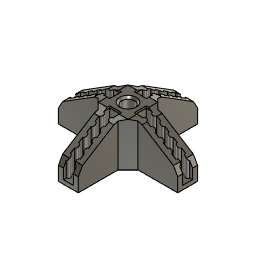
QuadAdapters4 (Autodesk Fusion 360 design; units mm, degrees)
Autodesk Fusion 360 part; units mm, degrees
sketch "Sketch1" plane through (0, 0, 0) normal (0, 0, 1) x (1, 0, 0)
  line L0 (0, 0) -> (0, 50)
  line L1 (0, 50) -> (10, 50)
  line L2 (10, 50) -> (10, 0)
  line L3 (10, 0) -> (60, 0)
  line L4 (60, 0) -> (60, -10)
  line L5 (60, -10) -> (10, -10)
  line L6 (10, -10) -> (10, -60)
  line L7 (10, -60) -> (0, -60)
  line L8 (0, -60) -> (0, -10)
  line L9 (0, -10) -> (-50, -10)
  line L10 (-50, -10) -> (-50, 0)
  line L11 (-50, 0) -> (0, 0)
  line L12 (-5, 5) -> (-5, 55)
  line L13 (-5, 55) -> (15, 55)
  line L14 (15, 55) -> (15, 5)
  line L15 (15, 5) -> (65, 5)
  line L16 (65, 5) -> (65, -15)
  line L17 (65, -15) -> (15, -15)
  line L18 (15, -15) -> (15, -65)
  line L19 (15, -65) -> (-5, -65)
  line L20 (-5, -65) -> (-5, -15)
  line L21 (-5, -15) -> (-55, -15)
  line L22 (-55, -15) -> (-55, 5)
  line L23 (-55, 5) -> (-5, 5)
  line L24 (0, 55) -> (0, -65)
  line L25 (10, -65) -> (10, 55)
  line L26 (-55, 0) -> (65, 0)
  line L27 (65, -10) -> (-55, -10)
  circle A0 centre (0, 50) radius 2.1
  circle A1 centre (10, 50) radius 2.1
  circle A2 centre (0, 41.6667) radius 2.1
  circle A3 centre (10, 41.6667) radius 2.1
  circle A4 centre (0, 33.3333) radius 2.1
  circle A5 centre (10, 33.3333) radius 2.1
  circle A6 centre (0, 25) radius 2.1
  circle A7 centre (10, 25) radius 2.1
  circle A8 centre (0, 16.6667) radius 2.1
  circle A9 centre (10, 16.6667) radius 2.1
  circle A10 centre (0, 8.3333) radius 2.1
  circle A11 centre (10, 8.3333) radius 2.1
  circle A12 centre (0, 0) radius 2.1
  circle A13 centre (10, 0) radius 2.1
  line L28 (-68.0742, -5) -> (73.3109, -5)
  line L29 (5, 62.6678) -> (5, -70)
  circle A14 centre (0, -18.3333) radius 2.1
  circle A15 centre (10, -43.3333) radius 2.1
  line L30 (0, -60) -> (10, -60)
  circle A16 centre (0, -43.3333) radius 2.1
  circle A17 centre (0, -26.6667) radius 2.1
  line L31 (10, -60) -> (10, -10)
  circle A18 centre (0, -10) radius 2.1
  circle A19 centre (10, -35) radius 2.1
  circle A20 centre (0, -35) radius 2.1
  circle A21 centre (10, -51.6667) radius 2.1
  line L32 (0, -10) -> (0, -60)
  circle A22 centre (0, -51.6667) radius 2.1
  circle A23 centre (10, -26.6667) radius 2.1
  line L33 (-5, -15) -> (-5, -65)
  circle A24 centre (10, -10) radius 2.1
  circle A25 centre (0, -60) radius 2.1
  circle A26 centre (10, -18.3333) radius 2.1
  circle A27 centre (10, -60) radius 2.1
  circle A28 centre (-41.6667, -10) radius 2.1
  circle A29 centre (0, 0) radius 2.1
  circle A30 centre (-8.3333, -10) radius 2.1
  line L34 (-50, 0) -> (0, 0)
  circle A31 centre (-25, 0) radius 2.1
  circle A32 centre (-50, -10) radius 2.1
  circle A33 centre (-16.6667, -10) radius 2.1
  line L35 (-50, -10) -> (-50, 0)
  circle A34 centre (0, -10) radius 2.1
  circle A35 centre (-25, -10) radius 2.1
  circle A36 centre (-8.3333, 0) radius 2.1
  circle A37 centre (-33.3333, -10) radius 2.1
  circle A38 centre (-16.6667, 0) radius 2.1
  line L36 (0, -10) -> (-50, -10)
  circle A39 centre (-50, 0) radius 2.1
  circle A40 centre (-33.3333, 0) radius 2.1
  circle A41 centre (-41.6667, 0) radius 2.1
  line L37 (-55, -15) -> (-55, 5)
  circle A42 centre (10, -51.6667) radius 2.1
  circle A43 centre (0, -10) radius 2.1
  circle A44 centre (10, -18.3333) radius 2.1
  line L38 (0, -60) -> (0, -10)
  circle A45 centre (0, -35) radius 2.1
  circle A46 centre (10, -60) radius 2.1
  circle A47 centre (10, -26.6667) radius 2.1
  line L39 (10, -60) -> (0, -60)
  circle A48 centre (10, -10) radius 2.1
  circle A49 centre (10, -35) radius 2.1
  circle A50 centre (0, -18.3333) radius 2.1
  circle A51 centre (10, -43.3333) radius 2.1
  circle A52 centre (0, -26.6667) radius 2.1
  line L40 (10, -10) -> (10, -60)
  circle A53 centre (0, -60) radius 2.1
  circle A54 centre (0, -43.3333) radius 2.1
  circle A55 centre (0, -51.6667) radius 2.1
  line L41 (15, -65) -> (-5, -65)
  circle A56 centre (51.6667, 0) radius 2.1
  circle A57 centre (10, -10) radius 2.1
  circle A58 centre (18.3333, 0) radius 2.1
  line L42 (60, -10) -> (10, -10)
  circle A59 centre (35, -10) radius 2.1
  circle A60 centre (60, 0) radius 2.1
  circle A61 centre (26.6667, 0) radius 2.1
  line L43 (60, 0) -> (60, -10)
  circle A62 centre (10, 0) radius 2.1
  circle A63 centre (35, 0) radius 2.1
  circle A64 centre (18.3333, -10) radius 2.1
  circle A65 centre (43.3333, 0) radius 2.1
  circle A66 centre (26.6667, -10) radius 2.1
  line L44 (10, 0) -> (60, 0)
  circle A67 centre (60, -10) radius 2.1
  circle A68 centre (43.3333, -10) radius 2.1
  circle A69 centre (51.6667, -10) radius 2.1
  line L45 (65, 5) -> (65, -15)
  line L46 (0, 0) -> (-8.3333, 0)
  line L47 (-8.3333, 0) -> (-8.3333, -10)
  line L48 (-8.3333, -10) -> (0, -10)
  line L49 (0, -10) -> (0, 0)
  line L50 (18.3333, 0) -> (10, 0)
  line L51 (10, 0) -> (10, -10)
  line L52 (10, -10) -> (18.3333, -10)
  line L53 (18.3333, -10) -> (18.3333, 0)
  line L54 (0, 8.3333) -> (10, 8.3333)
  line L55 (10, 8.3333) -> (10, 0)
  line L56 (10, 0) -> (0, 0)
  line L57 (0, 0) -> (0, 8.3333)
  line L58 (0, -10) -> (10, -10)
  line L59 (10, -10) -> (10, -18.3333)
  line L60 (10, -18.3333) -> (0, -18.3333)
  line L61 (0, -18.3333) -> (0, -10)
  point P0 (0, -65)
  point P1 (10, -65)
  point P2 (0, -10)
  point P3 (0, -10)
  point P4 (5, -5)
  point P5 (0, -10)
  point P6 (-55, -10)
  point P7 (-5, 5)
  point P8 (-55, 0)
  point P9 (5, -5)
  point P10 (0, -10)
  point P11 (-5, -15)
  point P12 (10, -10)
  point P13 (10, -65)
  point P14 (-5, -15)
  point P15 (0, -65)
  point P16 (5, -5)
  point P17 (10, -10)
  point P18 (15, -15)
  point P19 (10, 0)
  point P20 (65, 0)
  point P21 (15, -15)
  point P22 (65, -10)
  point P23 (5, -5)
  point P24 (10, 0)
  point P25 (15, 5)
  dimension "d1" = 10
  dimension "d2" = 50
  dimension "d3" = 10
  dimension "d4" = 50
  dimension "d5" = 50
  dimension "d6" = -5
  dimension "d7" = 4.2
  dimension "d8" = 4.2
  dimension "d11" = 0
  dimension "d12" = -50
  dimension "d14" = 360
  constraint coincident L0.start L11.end
  constraint vertical L0
  constraint perpendicular L0 L1
  constraint perpendicular L1 L2
  constraint perpendicular L0 L3
  constraint perpendicular L3 L4
  constraint perpendicular L4 L5
  constraint perpendicular L5 L6
  constraint perpendicular L6 L7
  constraint perpendicular L7 L8
  constraint perpendicular L8 L9
  constraint perpendicular L7 L10
  constraint perpendicular L0 L11
  constraint coincident L13 L24.start
  constraint coincident L19 P15
  constraint perpendicular L19 L24
  constraint coincident L19 P13
  constraint coincident L13 L25.end
  constraint perpendicular L13 L25
  constraint coincident L22 P8
  constraint coincident L16 P20
  constraint perpendicular L16 L26
  constraint coincident L16 P22
  constraint coincident L22 P6
  constraint perpendicular L22 L27
  constraint coincident L0.end L1.start
  constraint coincident L1.end L2.start
  constraint perpendicular L22 L28
  constraint perpendicular L26 L29
  constraint symmetric L0.start L28 P10
  constraint symmetric L0.end L28 L7.end
  constraint symmetric L1.end L28 L6.end
  constraint symmetric P24 L28 P17
  constraint symmetric P7 L28 P11
  constraint symmetric L12.end L28 L19.end
  constraint symmetric L24.start L28 P15
  constraint symmetric L25.end L28 P13
  constraint symmetric A0 L28 A25
  constraint symmetric A1 L28 A27
  constraint symmetric A2 L28 A22
  constraint symmetric A3 L28 A21
  constraint symmetric A4 L28 A16
  constraint symmetric A5 L28 A15
  constraint symmetric A6 L28 A20
  constraint symmetric A7 L28 A19
  constraint symmetric A8 L28 A17
  constraint symmetric A9 L28 A23
  constraint symmetric A10 L28 A14
  constraint symmetric A11 L28 A26
  constraint symmetric A12 L28 A18
  constraint symmetric A13 L28 A24
  constraint coincident L28 P23
  constraint coincident L29 P23
  constraint horizontal L46
  constraint vertical L47
  constraint horizontal L48
  constraint vertical L49
  constraint coincident A30.centre L47.end
  constraint horizontal L50
  constraint vertical L51
  constraint horizontal L52
  constraint vertical L53
  constraint coincident P17 P12
  constraint coincident A58.centre L50.start
  constraint horizontal L54
  constraint vertical L55
  constraint horizontal L56
  constraint vertical L57
  constraint coincident P24 P19
  constraint coincident A10.centre L54.start
  constraint horizontal L58
  constraint vertical L59
  constraint horizontal L60
  constraint vertical L61
  constraint coincident A26.centre A44.centre
  measures "d1" distance of L0.end L1.end
  measures "d2" distance of P24 L3.end
  measures "d3" distance of L3.end L4.end
  measures "d4" distance of P17 L6.end
  measures "d5" distance of P5 L9.end
  measures "d7" diameter of A0
  measures "d8" diameter of A1
extrude "Extrude1" add sketch "Sketch1" along normal blind 45 contours L0 L11 L24 L26 A12 A29 L34 L46 L57 | L11 L24 L26 A12 A29 L34 L46 L49 | L24 L26 A12 A29 L49 L56 | L0 L24 L26 A12 A29 L56 L57 | L0 L11 L12 L13 L22 L23 L24 L26 A0 A2 A4 A6 A8 A10 A12 A29 L34 A31 A36 A38 A39 A40 A41 L37 L46 L57 | L0 L24 L26 A10 A12 L29 A29 L54 L56 L57 | L11 L24 L26 A12 L28 A29 L34 A36 L46 L47 L49 | L24 L26 A12 L28 L29 A29 L49 L56 | L0 L24 A10 L57 | L0 L24 A10 L54 L57 | L11 L26 L34 A36 L46 L47 | L11 L26 L34 A36 L46 | L24 L27 L28 L29 A18 A34 A43 L49 L58 | L9 L24 L27 L28 A18 A30 A34 L36 A43 L47 L48 L49 | L2 L25 L26 A11 A13 L29 A62 L54 L55 L56 | L25 L26 A13 L28 L29 A62 L51 L56 | L24 L27 A18 A34 A43 L49 L58 | L9 L24 L27 A18 A34 L36 A43 L48 L49 | L25 L27 L28 L29 A24 A48 A57 L51 L58 | L2 L25 L26 A13 A62 L55 L56 | L25 L26 A13 A62 L51 L56 | L0 L24 A8 | L0 L24 A8 | L11 L26 L34 A38 | L11 L26 L34 A38 | L8 L24 L27 A18 L32 A34 A43 L38 L58 L61 | L8 L9 L24 L27 A18 L32 A34 L36 A43 L38 L48 L61 | L8 L24 L27 L29 A14 A18 L32 A34 A43 L38 A50 L58 L60 L61 | L8 L9 L19 L20 L21 L22 L24 L27 A14 A16 A17 A18 A20 L32 A22 L33 A25 A28 A30 A32 A33 A34 A35 A37 L36 L37 A43 L38 A45 A50 A52 A53 A54 A55 L41 L48 L61 | L9 L27 A30 L36 L47 L48 | L5 L25 L27 L28 A24 A48 A57 L42 A64 L51 L52 L53 | L3 L25 L26 A13 L28 A58 A62 L44 L50 L51 L53 | L6 L25 L27 L29 L31 A24 A26 A44 A48 L40 A57 L58 L59 L60 | L2 L3 L25 L26 A13 A62 L44 L50 L55 | L3 L25 L26 A13 A62 L44 L50 L51 | L2 L3 L13 L14 L15 L16 L25 L26 A1 A3 A5 A7 A9 A11 A13 A56 A58 A60 A61 A62 A63 A65 L44 L45 L50 L55 | L2 L25 A11 L54 L55 | L9 L27 A30 L36 L48 | L9 L10 L27 A32 L35 L36 | L10 L27 A32 L35 | L10 L26 L35 A39 | L10 L11 L26 L34 L35 A39 | L5 L25 L27 A24 A48 A57 L42 L51 L52 | L25 L27 A24 A48 A57 L51 L58 | L6 L25 L27 L31 A24 A48 L40 A57 L58 L59 | L2 L25 A11 L55 | L0 L1 L24 A0 | L1 L24 A0 | L1 L25 A1 | L1 L2 L25 A1 | L0 L24 A6 | L0 L24 A6 | L11 L26 L34 A31 | L11 L26 L34 A31 | L8 L24 A14 L32 L38 A50 L60 L61 | L8 L24 A14 L32 L38 A50 L61 | L9 L27 A32 L36 | L11 L26 L34 A39 | L9 L27 A33 L36 | L9 L27 A33 L36 | L5 L6 L25 L27 L31 A24 A48 L40 A57 L42 L52 L59 | L5 L6 L16 L17 L18 L19 L25 L27 A15 L31 A19 A21 A23 A24 A26 A27 A42 A44 A46 A47 A48 A49 A51 L40 L41 A57 L42 A59 A64 A66 A67 A68 A69 L45 L52 L59 | L5 L27 L42 A64 L52 L53 | L3 L26 A58 L44 L50 L53 | L6 L25 L31 A26 A44 L40 L59 L60 | L3 L26 A58 L44 L50 | L0 L24 A0 | L2 L25 A1 | L2 L25 A9 | L2 L25 A9 | L9 L27 A28 L36 | L9 L27 A28 L36 | L11 L26 L34 A41 | L11 L26 L34 A41 | L5 L27 L42 A64 L52 | L3 L4 L26 A60 L43 L44 | L4 L26 A60 L43 | L4 L27 L43 A67 | L4 L5 L27 L42 L43 A67 | L6 L25 L31 A26 A44 L40 L59 | L6 L7 L25 L30 L31 A27 A46 L39 L40 | L7 L25 L30 A27 A46 L39 | L7 L24 L30 A25 L39 A53 | L7 L8 L24 L30 L32 A25 L38 L39 A53 | L0 L24 A2 | L0 L24 A2 | L2 L25 A3 | L2 L25 A3 | L0 L24 A4 | L0 L24 A4 | L11 L26 L34 A40 | L11 L26 L34 A40 | L8 L24 A17 L32 L38 A52 | L8 L24 A17 L32 L38 A52 | L9 L27 A35 L36 | L9 L27 A35 L36 | L3 L26 A60 L44 | L5 L27 L42 A67 | L5 L27 L42 A66 | L5 L27 L42 A66 | L3 L26 A61 L44 | L3 L26 A61 L44 | L6 L25 L31 A27 A46 L40 | L8 L24 L32 A25 L38 A53 | L6 L25 L31 A23 A47 L40 | L6 L25 L31 A23 A47 L40 | L2 L25 A7 | L2 L25 A7 | L9 L27 A37 L36 | L9 L27 A37 L36 | L3 L26 A56 L44 | L3 L26 A56 L44 | L5 L27 L42 A69 | L5 L27 L42 A69 | L6 L25 L31 A21 A42 L40 | L6 L25 L31 A21 A42 L40 | L8 L24 L32 A22 L38 A55 | L8 L24 L32 A22 L38 A55 | L2 L25 A5 | L2 L25 A5 | L8 L24 A20 L32 L38 A45 | L8 L24 A20 L32 L38 A45 | L5 L27 L42 A59 | L5 L27 L42 A59 | L3 L26 A63 L44 | L3 L26 A63 L44 | L6 L25 L31 A19 A49 L40 | L6 L25 L31 A19 A49 L40 | L3 L26 A65 L44 | L3 L26 A65 L44 | L5 L27 L42 A68 | L5 L27 L42 A68 | L6 L25 A15 L31 A51 L40 | L6 L25 A15 L31 A51 L40 | L8 L24 A16 L32 L38 A54 | L8 L24 A16 L32 L38 A54
extrude "Extrude2" add sketch "Sketch1" 5 faces at (0.5556, -5, 0) (0.5556, -5, 0) (0.5556, -5, 0) (0.5556, -5, 0) (0.5556, -5, 0) along normal blind 5
sketch "Sketch2" plane through (15, 0, 0) normal (1, 0, 0) x (0, 1, 0)
  line L0 (-15, 0) -> (-15, 45)
  line L1 (-15, 45) -> (-65, 45)
  line L2 (-65, 45) -> (-65, 0)
  line L3 (-65, 0) -> (-15, 0)
  line L4 (-25, 45) -> (-65, 20)
  line L5 (55, 0) -> (55, 45)
  line L6 (55, 45) -> (5, 45)
  line L7 (5, 45) -> (5, 0)
  line L8 (5, 0) -> (55, 0)
  line L9 (5, 45) -> (-15, 45)
  line L10 (-5, 45) -> (-5, 58.2647)
  line L11 (15, 45) -> (55, 20)
  point P0 (-15, 45)
  dimension "d19" = 20
  dimension "d20" = 10
  constraint coincident L1 L4.start
  constraint coincident L2 L4.end
  constraint coincident L6.end L7.start
  constraint coincident P0 L0.end
  constraint midpoint L9 L10.start
  constraint perpendicular L9 L10
  constraint symmetric L4.start L10 L11.start
  constraint symmetric L4.end L10 L11.end
  measures "d19" distance of L2.end L4.end
  measures "d20" distance of L4.start P0
extrude "Extrude3" cut sketch "Sketch2" against normal blind 80 contours L1 L2 L4
extrude "Extrude4" cut sketch "Sketch2" against normal blind 40 contours L5 L6 L11
sketch "Sketch3" plane through (0, 5, 0) normal (0, 1, 0) x (-1, 0, 0)
  line L0 (55, 0) -> (55, 45)
  line L1 (55, 45) -> (5, 45)
  line L2 (5, 45) -> (5, 0)
  line L3 (5, 0) -> (55, 0)
  line L4 (55, 20) -> (15, 45)
  line L5 (-15, 0) -> (-15, 45)
  line L6 (-15, 45) -> (-65, 45)
  line L7 (-65, 45) -> (-65, 0)
  line L8 (-65, 0) -> (-15, 0)
  line L9 (-15, 45) -> (5, 45)
  line L10 (-5, 45) -> (-5, 53.1094)
  line L11 (-65, 20) -> (-25, 45)
  point P0 (5, 45)
  dimension "d25" = 10
  dimension "d26" = 20
  constraint coincident L0 L4.start
  constraint coincident L1 L4.end
  constraint coincident L5.end L6.start
  constraint coincident P0 L1.end
  constraint midpoint L9 L10.start
  constraint perpendicular L9 L10
  constraint symmetric L4.start L10 L11.start
  constraint symmetric L4.end L10 L11.end
  measures "d25" distance of L4.end P0
  measures "d26" distance of L0.start L4.start
extrude "Extrude5" cut sketch "Sketch3" against normal blind 60 contours L0 L1 L4 | L6 L7 L11
sketch "Sketch4" plane through (0, 0, 45) normal (0, 0, 1) x (-1, 0, 0)
  line L0 (15, 8.7224) -> (15, 15)
  line L1 (15, 15) -> (5, 15)
  line L2 (5, 15) -> (5, 25)
  line L3 (5, 25) -> (-1.2776, 25)
  arc A0 (-1.2776, 25) -> (0, 24.5667) centre (0, 26.6667) ccw
  line L4 (0, 24.5667) -> (0, 18.3333)
  line L5 (0, 18.3333) -> (-10, 18.3333)
  line L6 (-10, 18.3333) -> (-10, 24.5667)
  arc A1 (-10, 24.5667) -> (-8.7224, 25) centre (-10, 26.6667) ccw
  line L7 (-8.7224, 25) -> (-15, 25)
  line L8 (-15, 25) -> (-15, 15)
  line L9 (-15, 15) -> (-25, 15)
  line L10 (-25, 15) -> (-25, 8.7224)
  arc A2 (-25, 8.7224) -> (-24.5667, 10) centre (-26.6667, 10) ccw
  line L11 (-24.5667, 10) -> (-18.3333, 10)
  line L12 (-18.3333, 10) -> (-18.3333, 0)
  line L13 (-18.3333, 0) -> (-24.5667, 0)
  arc A3 (-24.5667, 0) -> (-25, 1.2776) centre (-26.6667, 0) ccw
  line L14 (-25, 1.2776) -> (-25, -5)
  line L15 (-25, -5) -> (-15, -5)
  line L16 (-15, -5) -> (-15, -15)
  line L17 (-15, -15) -> (-8.7224, -15)
  arc A4 (-8.7224, -15) -> (-10, -14.5667) centre (-10, -16.6667) ccw
  line L18 (-10, -14.5667) -> (-10, -8.3333)
  line L19 (-10, -8.3333) -> (0, -8.3333)
  line L20 (0, -8.3333) -> (0, -14.5667)
  arc A5 (0, -14.5667) -> (-1.2776, -15) centre (0, -16.6667) ccw
  line L21 (-1.2776, -15) -> (5, -15)
  line L22 (5, -15) -> (5, -5)
  line L23 (5, -5) -> (15, -5)
  line L24 (15, -5) -> (15, 1.2776)
  arc A6 (15, 1.2776) -> (14.5667, 0) centre (16.6667, 0) ccw
  line L25 (14.5667, 0) -> (8.3333, 0)
  line L26 (8.3333, 0) -> (8.3333, 10)
  line L27 (8.3333, 10) -> (14.5667, 10)
  arc A7 (14.5667, 10) -> (15, 8.7224) centre (16.6667, 10) ccw
  line L28 (-18.3333, 5) -> (8.3333, 5)
  line L29 (-5, -8.3333) -> (-5, 18.3333)
  circle A8 centre (-5, 5) radius 6.5
  circle A9 centre (-5, 5) radius 1.75
  dimension "d29" = 13
  dimension "d30" = 3.5
  constraint midpoint L12 L28.start
  constraint midpoint L26 L28.end
  constraint midpoint L19 L29.start
  constraint midpoint L5 L29.end
  constraint midpoint L28 A8.centre
  constraint concentric A8 A9
  measures "d29" diameter of A8
  measures "d30" diameter of A9
extrude "Extrude6" cut sketch "Sketch4" against normal blind 75 contours L28 L29 A9 | L28 L29 A9 | L28 L29 A9 | L28 L29 A9
extrude "Extrude7" cut sketch "Sketch4" against normal blind 40 contours L28 L29 A8 A9 | L28 L29 A8 A9 | L28 L29 A8 A9 | L28 L29 A8 A9
chamfer "Chamfer1" distance 2 angle 45 1 edges at (11.0601, -7.3505, 45)
chamfer "Chamfer2" distance 5 angle 45 4 edges at (-55, -12.5, 20) (-55, 2.5, 20) (-15, 1.8612, 45) (-15, -11.8612, 45)
chamfer "Chamfer2" distance 5 angle 45 12 edges at (-2.5, -65, 20) (12.5, -65, 20) (-1.8612, -25, 45) (11.8612, -25, 45) (-1.8612, 15, 45) (11.8612, 15, 45) (12.5, 55, 20) (-2.5, 55, 20) (25, 1.8612, 45) (25, -11.8612, 45) (65, -12.5, 20) (65, 2.5, 20)
chamfer "Chamfer3" distance 10 angle 45 4 edges at (-5, -15, 22.5) (-5, 5, 22.5) (15, 5, 22.5) (15, -15, 22.5)
chamfer "Chamfer4" distance 1 angle 45 1 faces at (1.6667, -38.3333, 0)
chamfer "Chamfer5" distance 1 angle 45 12 edges at (5, -18.3333, 45) (0, -19.1667, 45) (10, -19.1667, 45) (-9.1667, -10, 45) (-8.3333, -5, 45) (-9.1667, 0, 45) (0, 9.1667, 45) (5, 8.3333, 45) (10, 9.1667, 45) (19.1667, 0, 45) (18.3333, -5, 45) (19.1667, -10, 45)
equation "d33 = -45.00 mm + 5 mm"
